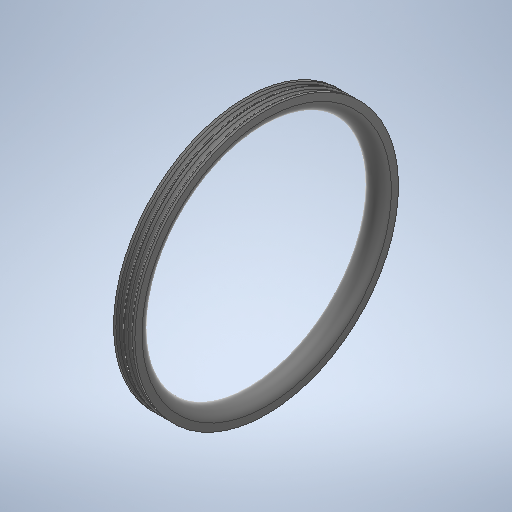
# Autodesk Inventor part: TPU Tire
Saved by Autodesk Inventor 2025.2 (Build 292293000, 293)
## iProperties
Created: 2025-01-18
Part Number: TPU Tire
Material: Generic
Document SubType Name: Modeling
Designer: mtidd
Density: 1 g/cm^3
Appearance: Default
Mass: 82.7029 g
Surface Area: 285.366 cm^2
Volume: 82.7029 cm^3
Author: mtidd
Autodesk Inventor part; units mm, degrees
ref_plane "YZ Plane" through (0, 0, 0) normal (1, 0, 0) x (0, 1, 0)
ref_plane "XZ Plane" through (0, 0, 0) normal (0, 1, 0) x (-1, 0, 0)
ref_plane "XY Plane" through (0, 0, 0) normal (0, 0, 1) x (1, 0, 0)
sketch "Sketch3" plane through (0, 0, 0) normal (0, 0, 1) x (1, 0, 0)
  arc A0 (-7.5, 7.5) -> (7.5, 7.5) centre (0, 7.5) ccw
  line L0 (0, -80) -> (50, -80)
  line L1 (0, -80) -> (50, -80) construction
  line L2 (-7.5, 7.5) -> (7.5, 7.5)
  line L3 (7.5, 7.5) -> (7.5, 12.5)
  line L4 (7.5, 12.5) -> (-7.5, 12.5)
  line L5 (-7.5, 12.5) -> (-7.5, 7.5)
  line L6 (-4.5, 12.5) -> (-1.5, 12.5)
  line L7 (-1.5, 12.5) -> (-1.5, 10.5)
  line L8 (-1.5, 10.5) -> (-4.5, 10.5)
  line L9 (-4.5, 10.5) -> (-4.5, 12.5)
  line L10 (1.5, 10.5) -> (4.5, 10.5)
  line L11 (4.5, 10.5) -> (4.5, 12.5)
  line L12 (4.5, 12.5) -> (1.5, 12.5)
  line L13 (1.5, 12.5) -> (1.5, 10.5)
  point P0 (0, 0)
  point P1 (7.5, 7.5)
  dimension "d34" = 0
  dimension "d51" = 5
  dimension "d52" = 3
  dimension "d53" = 2
  dimension "d54" = 3
  dimension "d55" = 2
  constraints: 28 end point, 6 parallel, 4 horizontal, 3 perpendicular, 3 point on circle, 2 point on line, 1 centre point, 1 collinear
  measures "d34" distance between parallel lines of L0 L1
  measures "d51" distance of L3.end L2.end
  measures "d52" distance of L7.end L8.end
  measures "d53" distance of L6.end L7.end
  measures "d54" distance of L12.end L11.end
  measures "d55" distance of L11.end L10.end
revolve "Revolution2" add sketch "Sketch3" angle 360 about axis through (0, -80, 0) along (1, 0, 0) contours L2 A0 | L5 L4 L9 L8 L7 L13 L10 L11 L3 L2
fillet "Fillet1" radius 1.5 8 edges at (-1.5, -170.5, 0) (1.5, -170.5, 0) (4.5, -170.5, 0) (-4.5, -170.5, 0) (-4.5, -172.5, 0) (-1.5, -172.5, 0) (1.5, -172.5, 0) (4.5, -172.5, 0)
body "Solid2"
